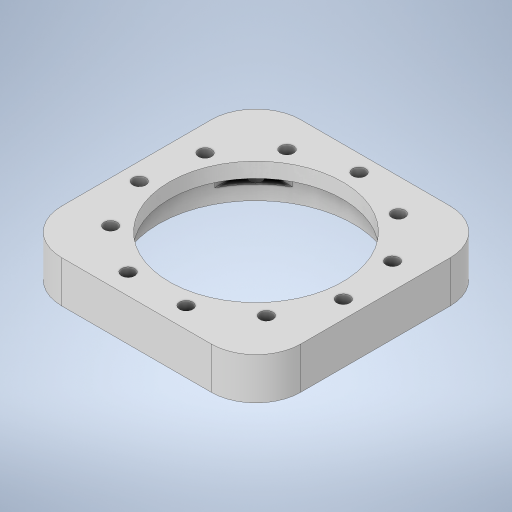
# Autodesk Inventor part: 사이클로이드 기어 하우징
Saved by Autodesk Inventor 2023 (Build 270158000, 158)
## iProperties
Created: 2022-06-19
Part Number: 사이클로이드 기어 하우징
Material: 일반
Document SubType Name: Modeling
Designer: fly01
Density: 1 g/cm^3
Appearance: 기본값
Author: fly01
Autodesk Inventor part; units mm, degrees
ref_plane "YZ Plane" through (0, 0, 0) normal (1, 0, 0) x (0, 1, 0)
ref_plane "XZ Plane" through (0, 0, 0) normal (0, 1, 0) x (-1, 0, 0)
ref_plane "XY Plane" through (0, 0, 0) normal (0, 0, 1) x (1, 0, 0)
sketch "스케치1" plane through (0, 0, 0) normal (0, 0, 1) x (1, 0, 0)
  line L0 (-25, -30) -> (25, -30) construction
  line L1 (30, -25) -> (30, 25) construction
  line L2 (25, 30) -> (-25, 30) construction
  line L3 (-30, 25) -> (-30, -25) construction
  line L4 (-30, -30) -> (30, 30) construction
  line L5 (30, -30) -> (-30, 30) construction
  arc A0 (-25, 30) -> (-30, 25) centre (-25, 25) ccw
  arc A1 (30, 25) -> (25, 30) centre (25, 25) ccw
  arc A2 (25, -30) -> (30, -25) centre (25, -25) ccw
  arc A3 (-30, -25) -> (-25, -30) centre (-25, -25) ccw
  circle A4 centre (0, 0) radius 7.5
  circle A5 centre (0, 0) radius 35 construction
  circle A6 centre (-24.7487, 24.7487) radius 2
  circle A7 centre (-24.7487, -24.7487) radius 2
  circle A8 centre (24.7487, -24.7487) radius 2
  circle A9 centre (24.7487, 24.7487) radius 2
  circle A10 centre (0, 0) radius 32.6
  circle A11 centre (0, 0) radius 25 construction
  line L6 (-25, 40) -> (25, 40)
  arc A12 (40, 25) -> (25, 40) centre (25, 25) ccw
  line L7 (40, 25) -> (40, -25)
  arc A13 (25, -40) -> (40, -25) centre (25, -25) ccw
  line L8 (25, -40) -> (-25, -40)
  arc A14 (-40, -25) -> (-25, -40) centre (-25, -25) ccw
  line L9 (-40, -25) -> (-40, 25)
  arc A15 (-25, 40) -> (-40, 25) centre (-25, 25) ccw
  dimension "d4" = 70
  dimension "d0" = 60
  dimension "d1" = 60
  dimension "d2" = 5
  dimension "d3" = 15
  dimension "d5" = 4
  dimension "d8" = 360
  dimension "d10" = 65.2
  dimension "d11" = 50
  dimension "d12" = 10
  constraints: 20 end point, 16 point on circle, 15 centre point, 9 point on line, 8 tangent, 4 coincident, 4 parallel, 3 equal radius, 2 midpoint, 2 perpendicular, 1 horizontal, 19 other
  measures "d0" distance of L5.end L4.end
  measures "d1" distance of L4.end L5.start
  measures "d2" radius of A0
  measures "d3" diameter of A4
  measures "d5" diameter of A6
  measures "d10" diameter of A10
  measures "d11" diameter of A11
  measures "d12" distance between parallel lines of L2 L6
extrude "돌출1" add sketch "스케치1" along normal blind 9 contours L6 A12 L7 A13 L8 A14 L9 A15
sketch "스케치2" plane through (0, 0, 0) normal (0, 0, -1) x (-1, 0, 0)
  line L0 (25, -40) -> (-25, -40) projected
  arc A0 (25, -40) -> (40, -25) centre (25, -25) ccw projected
  line L1 (40, 25) -> (40, -25) projected
  arc A1 (40, 25) -> (25, 40) centre (25, 25) ccw projected
  line L2 (-25, 40) -> (25, 40) projected
  arc A2 (-25, 40) -> (-40, 25) centre (-25, 25) ccw projected
  line L3 (-40, -25) -> (-40, 25) projected
  arc A3 (-40, -25) -> (-25, -40) centre (-25, -25) ccw projected
  circle A4 centre (0, 0) radius 32.6 construction
  circle A5 centre (-24.7487, 24.7487) radius 2 projected
  circle A6 centre (-24.7487, -24.7487) radius 2 projected
  circle A7 centre (24.7487, -24.7487) radius 2 projected
  circle A8 centre (24.7487, 24.7487) radius 2 projected
  circle A9 centre (0, 0) radius 29
  dimension "d15" = 58
  constraints: 1 centre point, 1 coincident
  measures "d15" diameter of A9
extrude "돌출2" add sketch "스케치2" along normal blind 5 contours L0 A3 L3 A2 L2 A1 L1 A0 | A5 | A6 | A7 | A8
sketch "스케치9" plane through (0, 0, 0) normal (0, 0, 1) x (1, 0, 0)
  circle A0 centre (-24.7487, 24.7487) radius 2 projected
  line L0 (-28.9057, 24.7487) -> (-26.8272, 28.3487)
  line L1 (-26.8272, 28.3487) -> (-22.6703, 28.3487)
  line L2 (-22.6703, 28.3487) -> (-20.5918, 24.7487)
  line L3 (-20.5918, 24.7487) -> (-22.6703, 21.1487)
  line L4 (-22.6703, 21.1487) -> (-26.8272, 21.1487)
  line L5 (-26.8272, 21.1487) -> (-28.9057, 24.7487)
  line L6 (-28.9057, 24.7487) -> (-28.9057, 15.0739)
  circle A1 centre (0, 0) radius 32.6 projected
  line L7 (-22.6703, 28.3487) -> (-16.0969, 28.3487)
  point P0 (-20.7972, 25.1045)
  point P1 (-24.8091, 21.1487)
  dimension "d27" = 7.2
  constraints: 16 end point, 2 point on circle, 1 coincident, 1 horizontal, 1 vertical, 13 other
  measures "d27" distance between parallel lines of L1 L4
extrude "돌출4" cut sketch "스케치9" along normal blind 4.2 contours L0 L1 L2 A1 L4 L5 | L5 L4 A1 L6 | L7 A1 L2 | A1 L2 L3 L4 picked at (-21.824, 23.2537)
mirror "미러1" about plane through (0, 0, 0) normal (0, 1, 0) of "돌출4"
mirror "미러2" about plane through (0, 0, 0) normal (1, 0, 0) of "돌출4", "미러1"
sketch "스케치10" plane through (0, 0, -5) normal (0, 0, -1) x (-1, 0, 0)
  circle A0 centre (0, 0) radius 32.5 construction
  circle A1 centre (0, -34.5) radius 2 construction
  circle A2 centre (0, -34.5) radius 2.2
  dimension "d30" = 65
  dimension "d31" = 4
  dimension "d32" = 0.2
  constraints: 3 centre point, 1 coincident, 1 tangent
  measures "d30" diameter of A0
  measures "d31" diameter of A1
  measures "d32" radial gap between concentric circles of A1 A2
extrude "돌출5" cut sketch "스케치10" against normal blind 5
pattern_circular "원형 패턴1" count 11 over 360 about axis through (0, 0, 0) along (0, 0, -1) of "돌출5"
